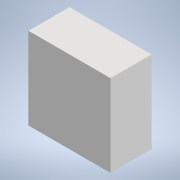
# Autodesk Inventor part: tieRod
Saved by Autodesk Inventor 2020.2 (Build 242310000, 310)
## iProperties
Created: 2020-01-21
Part Number: tieRod
Material: Generic
Document SubType Name: Modeling
Designer: robst
Density: 1 g/cm^3
Appearance: Default
Author: robst
Autodesk Inventor part; units mm, degrees
ref_plane "YZ Plane" through (0, 0, 0) normal (1, 0, 0) x (0, 1, 0)
ref_plane "XZ Plane" through (0, 0, 0) normal (0, 1, 0) x (-1, 0, 0)
ref_plane "XY Plane" through (0, 0, 0) normal (0, 0, 1) x (1, 0, 0)
sketch "Sketch1" plane through (0, 0, 0) normal (0, 0, 1) x (1, 0, 0)
  line L0 (-19.05, -12.7) -> (19.05, -12.7)
  line L1 (19.05, -12.7) -> (19.05, 12.7)
  line L2 (19.05, 12.7) -> (-19.05, 12.7)
  line L3 (-19.05, 12.7) -> (-19.05, -12.7)
  line L4 (-19.05, -12.7) -> (19.05, 12.7) construction
  line L5 (19.05, -12.7) -> (-19.05, 12.7) construction
  point P0 (0, 0)
  dimension "d0" = 38.1
  dimension "d1" = 25.4
  constraints: 12 end point, 2 midpoint, 2 parallel, 1 horizontal, 1 perpendicular
  measures "d0" distance of L0.start L0.end
  measures "d1" distance of L2.end L0.start
extrude "Extrusion1" add sketch "Sketch1" against normal blind 12.7
sketch "Sketch2" plane through (-19.05, -12.7, 0) normal (-1, 0, 0) x (0, 0, 1)
  line L0 (-12.7, 0) -> (-12.7, 25.4) construction
  line L1 (0, 25.4) -> (0, 0) construction
  line L2 (-12.7, 25.4) -> (0, 0) construction
  line L3 (0, 25.4) -> (-12.7, 0) construction
  circle A0 centre (-6.35, 12.7) radius 3.683
  point P0 (0, 12.7)
  dimension "d4" = 7.366
  constraints: 4 end point, 1 centre point, 1 midpoint
  measures "d4" diameter of A0
extrude "Extrusion2" cut sketch "Sketch2" against normal blind 12.7
sketch "Sketch3" plane through (0, 0, 0) normal (0, 0, 1) x (1, 0, 0)
  circle A0 centre (0, 0) radius 5.2705
  dimension "d7" = 10.541
  constraints: 1 centre point, 1 coincident
  measures "d7" diameter of A0
extrude "Extrusion3" cut sketch "Sketch3" against normal through all
body "Solid1"
